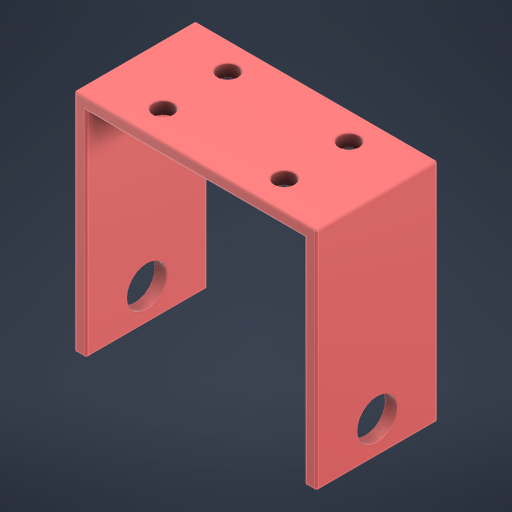
# Autodesk Inventor part: HOLDER
Saved by Autodesk Inventor 2023 (Build 270158000, 158)
## iProperties
Created: 2023-12-28
Part Number: HOLDER
Material: Steel, Alloy
Document SubType Name: Modeling
Designer: User
Density: 7.73 g/cm^3
Appearance: Smooth - Red
Author: User
Autodesk Inventor part; units mm, degrees
ref_plane "YZ Plane" through (0, 0, 0) normal (1, 0, 0) x (0, 1, 0)
ref_plane "XZ Plane" through (0, 0, 0) normal (0, 1, 0) x (-1, 0, 0)
ref_plane "XY Plane" through (0, 0, 0) normal (0, 0, 1) x (1, 0, 0)
sketch "Sketch1" plane through (0, 0, 0) normal (0, 0, 1) x (1, 0, 0)
  line L0 (27, 28) -> (27, -25)
  line L1 (27, -25) -> (-27, -25)
  line L2 (-27, -25) -> (-27, 28)
  line L3 (-30, 28) -> (-30, -28)
  line L4 (-30, -28) -> (30, -28)
  line L5 (30, -28) -> (30, 28)
  line L6 (30, 28) -> (27, 28)
  line L7 (-27, 28) -> (-30, 28)
  point P0 (0, 0)
  dimension "d4" = 56
  dimension "d5" = 53
  constraints: 16 end point, 4 parallel, 2 perpendicular
  measures "d4" distance of L3.start L3.end
  measures "d5" distance of L1.end L2.end
extrude "Extrusion1" add sketch "Sketch1" along normal blind 30
sketch "Sketch2" plane through (-27, -25, 0) normal (1, 0, 0) x (0, 0, -1)
  line L0 (0, 0) -> (-30, 0) projected
  line L1 (0, 0) -> (0, 53) projected
  point P0 (0, 25)
  point P1 (-15, 45)
  dimension "d8" = 45
  dimension "d9" = 15
  measures "d8" distance from line of L0 point (-15, 45)
  measures "d9" distance from line of L1 point (-15, 45)
hole "Hole1" at (-27, 20, 15) direction (-1, 0, 0) diameter 10 end through all
sketch "Sketch3" plane through (30, -28, 0) normal (1, 0, 0) x (0, 0, -1)
  line L0 (0, 3) -> (-30, 3) projected
  line L1 (-30, 0) -> (-30, 56) projected
  point P0 (0, 28)
  point P1 (-15, 48)
  dimension "d17" = 45
  dimension "d18" = 15
  measures "d17" distance from line of L0 point (-15, 48)
  measures "d18" distance from line of L1 point (-15, 48)
hole "Hole2" at (30, 20, 15) direction (-1, 0, 0) diameter 10 end through all
sketch "Sketch4" plane through (-30, -28, 0) normal (0, -1, 0) x (1, 0, 0)
  line L0 (0, 0) -> (60, 0) projected
  line L1 (60, 0) -> (60, 30) projected
  line L2 (0, 30) -> (60, 30) projected
  line L3 (0, 0) -> (0, 30) projected
  point P0 (30, 0)
  point P1 (45, 7)
  point P2 (45, 23)
  point P3 (15, 7)
  point P4 (15, 23)
  dimension "d26" = 7
  dimension "d27" = 15
  dimension "d28" = 7
  dimension "d29" = 15
  dimension "d30" = 7
  dimension "d31" = 15
  dimension "d32" = 15
  dimension "d33" = 7
  measures "d26" distance from line of L0 point (45, 7)
  measures "d27" distance from line of L1 point (45, 7)
  measures "d28" distance from line of L2 point (45, 23)
  measures "d29" distance from line of L1 point (45, 23)
  measures "d30" distance from line of L0 point (15, 7)
  measures "d31" distance from line of L3 point (15, 7)
  measures "d32" distance from line of L3 point (15, 23)
  measures "d33" distance from line of L2 point (15, 23)
hole "Hole3" at (15, -28, 23) at (15, -28, 7) at (-15, -28, 7) at (-15, -28, 23) direction (0, 1, 0) diameter 5 end through all
fillet "Fillet1" radius 0.5 21 edges at (30, -28, 15) (30, 0, 0) (27, 1.5, 0) (0, -25, 0) (0, -28, 0) (30, 0, 30) (30, 28, 15) (0, -28, 30) (-30, -28, 15) (-27, 1.5, 0) (-27, 28, 15) (-30, 28, 15) (-30, 0, 0) (-27, 1.5, 30) (-30, 0, 30) (27, 1.5, 30) (27, 28, 15) (28.5, 28, 0) (28.5, 28, 30) (-28.5, 28, 0) (-28.5, 28, 30)
body "Solid1"
